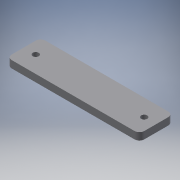
# Autodesk Inventor part: HeadSlide
Saved by Autodesk Inventor 2018 (Build 220112000, 112)
## iProperties
Created: 2018-01-01
Part Number: HeadSlide
Material: Generic
Document SubType Name: Modeling
Designer: reide
Density: 1 g/cm^3
Appearance: Default
Author: reide
Autodesk Inventor part; units mm, degrees
ref_plane "YZ Plane" through (0, 0, 0) normal (1, 0, 0) x (0, 1, 0)
ref_plane "XZ Plane" through (0, 0, 0) normal (0, 1, 0) x (-1, 0, 0)
ref_plane "XY Plane" through (0, 0, 0) normal (0, 0, 1) x (1, 0, 0)
sketch "Sketch1" plane through (0, 0, 0) normal (0, 0, 1) x (1, 0, 0)
  arc A0 (-89.3851, 275.0837) -> (-93.3851, 275.0837) centre (-91.3851, 275.0837) ccw projected
  line L0 (-89.3851, 275.0837) -> (-89.3851, 230.0837) projected
  arc A1 (-93.3851, 230.0837) -> (-89.3851, 230.0837) centre (-91.3851, 230.0837) ccw projected
  line L1 (-93.3851, 230.0837) -> (-93.3851, 275.0837) projected
  arc A2 (-44.3851, 275.0837) -> (-48.3851, 275.0837) centre (-46.3851, 275.0837) ccw projected
  line L2 (-44.3851, 275.0837) -> (-44.3851, 230.0837) projected
  arc A3 (-48.3851, 230.0837) -> (-44.3851, 230.0837) centre (-46.3851, 230.0837) ccw projected
  line L3 (-48.3851, 230.0837) -> (-48.3851, 275.0837) projected
  circle A4 centre (-6.132, -79.3472) radius 1.25 projected
  circle A5 centre (-145.3842, 185.8247) radius 1.5 projected
  circle A6 centre (-153.8932, -1.3222) radius 1.5 projected
  circle A7 centre (-145.3842, -79.3472) radius 1.5 projected
  circle A8 centre (-129.8902, 6.8528) radius 1.5 projected
  circle A9 centre (-116.3012, -71.1722) radius 1.5 projected
  circle A10 centre (-129.8902, 272.0247) radius 1.5 projected
  circle A11 centre (-129.8902, 185.8247) radius 1.5 projected
  circle A12 centre (-116.3012, 263.8497) radius 1.5 projected
  circle A13 centre (17.871, -71.1722) radius 1.5 projected
  circle A14 centre (-6.132, 6.8528) radius 1.5 projected
  circle A15 centre (-19.721, -1.3222) radius 1.5 projected
  circle A16 centre (17.871, 263.8497) radius 1.5 projected
  circle A17 centre (9.362, 272.0247) radius 1.5 projected
  circle A18 centre (9.362, 185.8247) radius 1.5 projected
  circle A19 centre (-19.721, 193.9997) radius 1.5 projected
  circle A20 centre (-19.721, 263.8497) radius 1.5 projected
  circle A21 centre (-6.132, 185.8247) radius 1.5 projected
  circle A22 centre (-6.132, 272.0247) radius 1.5 projected
  circle A23 centre (17.871, 193.9997) radius 1.5 projected
  circle A24 centre (-19.721, -71.1722) radius 1.5 projected
  circle A25 centre (9.362, -79.3472) radius 1.5 projected
  circle A26 centre (9.362, 6.8528) radius 1.5 projected
  circle A27 centre (17.871, -1.3222) radius 1.5 projected
  circle A28 centre (-116.3012, 193.9997) radius 1.5 projected
  circle A29 centre (-153.8932, 193.9997) radius 1.5 projected
  circle A30 centre (-153.8932, 263.8497) radius 1.5 projected
  circle A31 centre (-145.3842, 6.8528) radius 1.5 projected
  circle A32 centre (-129.8902, -79.3472) radius 1.5 projected
  circle A33 centre (-153.8932, -71.1722) radius 1.5 projected
  circle A34 centre (-116.3012, -1.3222) radius 1.5 projected
  circle A35 centre (-145.3842, 272.0247) radius 1.5 projected
  arc A36 (81.2372, 206.8201) -> (56.4499, 266.1206) centre (-44.5185, 189.0856) ccw projected
  ellipse E0 centre (-68.0111, 96.3387) end of major axis (-68.0111, -141.4053) minor radius 177.8 (56.4499, 266.1206) -> (-192.4721, 266.1206) ccw projected
  arc A37 (-192.4721, 266.1206) -> (-217.2594, 206.8201) centre (-91.5037, 189.0856) ccw projected
  arc A38 (-217.2594, 206.8201) -> (-217.2594, -14.1426) centre (566.1677, 96.3387) ccw projected
  arc A39 (-217.2594, -14.1426) -> (-192.4721, -73.4431) centre (-91.5037, 3.5918) ccw projected
  ellipse E1 centre (-68.0111, 96.3387) end of major axis (-68.0111, -141.4053) minor radius 177.8 (-192.4721, -73.4431) -> (56.4499, -73.4431) ccw projected
  arc A40 (56.4499, -73.4431) -> (81.2372, -14.1426) centre (-44.5185, 3.5918) ccw projected
  arc A41 (81.2372, -14.1426) -> (81.2372, 206.8201) centre (-702.1899, 96.3387) ccw projected
  circle A42 centre (-36.4956, 248.9087) radius 1.25 projected
  circle A43 centre (-101.2746, 318.7587) radius 1.25 projected
  circle A44 centre (-101.2746, 248.9087) radius 1.25 projected
  circle A45 centre (-36.4956, 318.7587) radius 1.25 projected
  circle A46 centre (-77.2861, -128.5803) radius 1.25 projected
  circle A47 centre (-92.2681, -54.079) radius 1.25 projected
  circle A48 centre (-53.9141, -54.079) radius 1.25 projected
  circle A49 centre (-58.7361, -128.5803) radius 1.25 projected
  line L4 (-82.971, -17.5241) -> (-82.971, 43.3967) projected
  line L5 (-82.971, 43.3967) -> (-52.491, 43.3967) projected
  line L6 (-52.491, 43.3967) -> (-52.491, -17.5241) projected
  line L7 (-52.491, -17.5241) -> (-82.971, -17.5241) projected
  circle A50 centre (-68.0111, 137.616) radius 35 projected
  line L8 (-123.7158, 171.3631) -> (-119.7158, 171.3631) projected
  arc A51 (-119.7158, 168.3632) -> (-119.7158, 171.3631) centre (-119.7158, 169.8631) ccw projected
  line L9 (-119.7158, 168.3632) -> (-123.7158, 168.3632) projected
  arc A52 (-123.7158, 171.3631) -> (-123.7158, 168.3632) centre (-123.7158, 169.8631) ccw projected
  line L10 (-123.6698, 106.6744) -> (-119.6698, 106.6744) projected
  arc A53 (-119.6698, 103.6746) -> (-119.6698, 106.6744) centre (-119.6698, 105.1745) ccw projected
  line L11 (-119.6698, 103.6746) -> (-123.6698, 103.6746) projected
  arc A54 (-123.6698, 106.6744) -> (-123.6698, 103.6746) centre (-123.6698, 105.1745) ccw projected
  line L12 (-9.1669, 171.4444) -> (-5.1669, 171.4444) projected
  arc A55 (-5.1669, 168.4446) -> (-5.1669, 171.4444) centre (-5.1669, 169.9445) ccw projected
  line L13 (-5.1669, 168.4446) -> (-9.1669, 168.4446) projected
  arc A56 (-9.1669, 171.4444) -> (-9.1669, 168.4446) centre (-9.1669, 169.9445) ccw projected
  line L14 (-5.1669, 103.6742) -> (-9.1669, 103.6742) projected
  arc A57 (-9.1669, 106.6741) -> (-9.1669, 103.6742) centre (-9.1669, 105.1742) ccw projected
  line L15 (-9.1669, 106.6741) -> (-5.1669, 106.6741) projected
  arc A58 (-5.1669, 103.6742) -> (-5.1669, 106.6741) centre (-5.1669, 105.1742) ccw projected
  arc A59 (-34.0816, 86.6493) -> (-37.0792, 86.6494) centre (-35.5804, 86.6492) ccw projected
  line L16 (-34.0816, 86.6493) -> (-34.0814, 82.6493) projected
  arc A60 (-37.0794, 82.6493) -> (-34.0814, 82.6493) centre (-35.5804, 82.6492) ccw projected
  line L17 (-37.0794, 82.6493) -> (-37.0792, 86.6494) projected
  arc A61 (-34.0865, 201.0395) -> (-37.0841, 201.0395) centre (-35.5853, 201.0395) ccw projected
  line L18 (-34.0865, 201.0395) -> (-34.0863, 197.0396) projected
  arc A62 (-37.0843, 197.0395) -> (-34.0863, 197.0396) centre (-35.5853, 197.0395) ccw projected
  line L19 (-37.0843, 197.0395) -> (-37.0841, 201.0395) projected
  arc A63 (-34.0812, 78.9993) -> (-37.0788, 78.9992) centre (-35.58, 78.9992) ccw projected
  line L20 (-34.0812, 78.9993) -> (-34.081, 74.9993) projected
  arc A64 (-37.079, 74.9993) -> (-34.081, 74.9993) centre (-35.58, 74.9992) ccw projected
  line L21 (-37.079, 74.9993) -> (-37.0788, 78.9992) projected
  arc A65 (-98.9325, 193.3865) -> (-101.9301, 193.3866) centre (-100.4313, 193.3865) ccw projected
  line L22 (-98.9325, 193.3865) -> (-98.9323, 189.3866) projected
  arc A66 (-101.9303, 189.3866) -> (-98.9323, 189.3866) centre (-100.4313, 189.3865) ccw projected
  line L23 (-101.9303, 189.3866) -> (-101.9301, 193.3866) projected
  circle A67 centre (-95.163, -4.4165) radius 1.25 projected
  circle A68 centre (-36.616, 37.0467) radius 1.25 projected
  circle A69 centre (-46.141, -14.3491) radius 1.25 projected
  circle A70 centre (-36.616, -11.1741) radius 1.25 projected
  circle A71 centre (-36.616, 12.9421) radius 1.25 projected
  circle A72 centre (-46.141, 40.2217) radius 1.25 projected
  circle A73 centre (-95.163, 40.4375) radius 1.25 projected
  arc A74 (-98.8512, 78.9533) -> (-101.8488, 78.9533) centre (-100.35, 78.9533) ccw projected
  line L24 (-98.8512, 78.9533) -> (-98.851, 74.9533) projected
  arc A75 (-101.849, 74.9533) -> (-98.851, 74.9533) centre (-100.35, 74.9533) ccw projected
  line L25 (-101.849, 74.9533) -> (-101.8488, 78.9533) projected
  line L26 (-34.0865, 193.3895) -> (-34.0863, 189.3896) projected
  arc A76 (-37.0843, 189.3896) -> (-34.0863, 189.3896) centre (-35.5853, 189.3895) ccw projected
  line L27 (-37.0843, 189.3896) -> (-37.0841, 193.3896) projected
  arc A77 (-34.0865, 193.3895) -> (-37.0841, 193.3896) centre (-35.5853, 193.3895) ccw projected
  arc A78 (-98.9379, 201.0395) -> (-101.9362, 200.9947) centre (-100.4367, 200.9934) ccw projected
  line L28 (-98.9379, 201.0395) -> (-98.9377, 196.9935) projected
  arc A79 (-101.9357, 196.9932) -> (-98.9377, 196.9935) centre (-100.4367, 196.9934) ccw projected
  line L29 (-101.9357, 196.9932) -> (-101.9362, 200.9947) projected
  arc A80 (-98.8567, 86.6032) -> (-101.8543, 86.6033) centre (-100.3555, 86.6032) ccw projected
  line L30 (-98.8567, 86.6032) -> (-98.8565, 82.6033) projected
  arc A81 (-101.8544, 82.6033) -> (-98.8565, 82.6033) centre (-100.3555, 82.6032) ccw projected
  line L31 (-101.8544, 82.6033) -> (-101.8543, 86.6033) projected
  line L32 (-16.8169, 106.6744) -> (-12.8169, 106.6744) projected
  arc A82 (-12.8169, 103.6746) -> (-12.8169, 106.6744) centre (-12.8169, 105.1745) ccw projected
  line L33 (-12.8169, 103.6746) -> (-16.8169, 103.6746) projected
  arc A83 (-16.8169, 106.6744) -> (-16.8169, 103.6746) centre (-16.8169, 105.1745) ccw projected
  line L34 (-16.8629, 171.439) -> (-12.8629, 171.439) projected
  arc A84 (-12.8629, 168.4391) -> (-12.8629, 171.439) centre (-12.8629, 169.9391) ccw projected
  line L35 (-12.8629, 168.4391) -> (-16.8629, 168.4391) projected
  arc A85 (-16.8629, 171.439) -> (-16.8629, 168.4391) centre (-16.8629, 169.9391) ccw projected
  line L36 (-131.3198, 106.6744) -> (-127.3198, 106.6744) projected
  arc A86 (-127.3198, 103.6746) -> (-127.3198, 106.6744) centre (-127.3198, 105.1745) ccw projected
  line L37 (-127.3198, 103.6746) -> (-131.3198, 103.6746) projected
  arc A87 (-131.3198, 106.6744) -> (-131.3198, 103.6746) centre (-131.3198, 105.1745) ccw projected
  line L38 (-131.3658, 171.3576) -> (-127.3658, 171.3576) projected
  arc A88 (-127.3658, 168.3578) -> (-127.3658, 171.3576) centre (-127.3658, 169.8577) ccw projected
  line L39 (-127.3658, 168.3578) -> (-131.3658, 168.3578) projected
  arc A89 (-131.3658, 171.3576) -> (-131.3658, 168.3578) centre (-131.3658, 169.8577) ccw projected
  circle A90 centre (-46.3851, 275.0837) radius 1.25 projected
  circle A91 centre (-91.3851, 275.0837) radius 1.25 projected
  line L40 (-41.3851, 222.0837) -> (-41.3851, 377.0837) projected
  line L41 (-96.3851, 377.0837) -> (-96.3851, 222.0837) projected
  line L42 (-46.3851, 275.0837) -> (-41.3851, 275.0837)
  line L43 (-41.3851, 275.0837) -> (-41.3851, 268.0837)
  line L44 (-41.3851, 268.0837) -> (-41.3851, 282.0837)
  line L45 (-41.3851, 282.0837) -> (-96.3851, 282.0837)
  line L46 (-41.3851, 274.0837) -> (-41.3851, 282.0837)
  line L47 (-41.3851, 282.0837) -> (-96.3851, 282.0837)
  line L48 (-96.3851, 282.0837) -> (-96.3851, 270.0837)
  line L49 (-41.3851, 270.0837) -> (-41.3851, 282.0837)
  line L50 (-41.3851, 282.0837) -> (-96.3851, 282.0837)
  line L51 (-96.3851, 282.0837) -> (-96.3851, 268.0837)
  line L52 (-96.3851, 268.0837) -> (-41.3851, 268.0837)
  line L53 (-41.3851, 268.0837) -> (-41.3851, 282.0837)
  point P0 (0, 0)
  dimension "d0" = 7
  dimension "d1" = 14
  constraints: 24 end point, 5 point on line, 4 horizontal, 3 parallel, 2 perpendicular, 2 other
  measures "d0" distance of L42.end L43.end
  measures "d1" distance of L43.end L44.end
extrude "Extrusion1" add sketch "Sketch1" along normal blind 3 contours L0 L52 L1 A0 | A0 L1 L52 L41 L45 L40 L42 A2 L3 L0 | L3 A2 L2 L52 | L2 L42 L40 L52
fillet "Fillet1" radius 2 4 edges at (-96.3851, 282.0837, 1.5) (-96.3851, 268.0837, 1.5) (-41.3851, 268.0837, 1.5) (-41.3851, 282.0837, 1.5)
body "Solid1"
